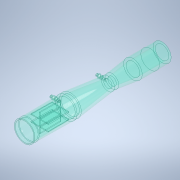
# Autodesk Inventor part: venturiwiwi
Saved by Autodesk Inventor 2020.2 (Build 242310000, 310)
## iProperties
Created: 2020-05-05
Part Number: venturiwiwi
Material: Generic
Document SubType Name: Modeling
Designer: JK
Density: 1 g/cm^3
Appearance: Indoor Pool
Author: JK
Autodesk Inventor part; units mm, degrees
sketch "Sketch1" plane through (0, 0, 0) normal (0, 1, 0) x (-1, 0, 0)
  line L0 (-5, 2.5) -> (5, 2.5)
  line L1 (5, 2.5) -> (5, -2.5)
  line L2 (5, -2.5) -> (-5, -2.5)
  line L3 (-5, -2.5) -> (-5, 2.5)
  line L4 (-5, 2.5) -> (5, -2.5) construction
  line L5 (5, 2.5) -> (-5, -2.5) construction
  line L6 (10.75, 52.5) -> (-10.75, 52.5)
  line L7 (-10.75, 52.5) -> (-10.75, 47.5)
  line L8 (-10.75, 47.5) -> (10.75, 47.5)
  line L9 (10.75, 47.5) -> (10.75, 52.5)
  line L10 (10.75, 52.5) -> (-10.75, 47.5) construction
  line L11 (-10.75, 52.5) -> (10.75, 47.5) construction
  line L12 (10.75, 47.5) -> (5, 2.5)
  line L13 (-10.75, 47.5) -> (-5, 2.5)
  line L14 (-13.75, 52.5) -> (13.75, 52.5)
  line L15 (13.75, 52.5) -> (13.75, 47.5)
  line L16 (13.75, 47.5) -> (-13.75, 47.5)
  line L17 (-13.75, 47.5) -> (-13.75, 52.5)
  line L18 (-13.75, 52.5) -> (13.75, 47.5) construction
  line L19 (13.75, 52.5) -> (-13.75, 47.5) construction
  line L20 (-8, 2.5) -> (8, 2.5)
  line L21 (8, 2.5) -> (8, -2.5)
  line L22 (8, -2.5) -> (-8, -2.5)
  line L23 (-8, -2.5) -> (-8, 2.5)
  line L24 (-8, 2.5) -> (8, -2.5) construction
  line L25 (8, 2.5) -> (-8, -2.5) construction
  line L26 (13.75, 47.5) -> (8, 2.5)
  line L27 (-13.75, 47.5) -> (-8, 2.5)
  line L28 (11.15, -27.5) -> (-11.15, -27.5)
  line L29 (-11.15, -27.5) -> (-11.15, -32.5)
  line L30 (-11.15, -32.5) -> (11.15, -32.5)
  line L31 (11.15, -32.5) -> (11.15, -27.5)
  line L32 (11.15, -27.5) -> (-11.15, -32.5) construction
  line L33 (-11.15, -27.5) -> (11.15, -32.5) construction
  line L34 (-8.15, -27.5) -> (8.15, -27.5)
  line L35 (8.15, -27.5) -> (8.15, -32.5)
  line L36 (8.15, -32.5) -> (-8.15, -32.5)
  line L37 (-8.15, -32.5) -> (-8.15, -27.5)
  line L38 (-8.15, -27.5) -> (8.15, -32.5) construction
  line L39 (8.15, -27.5) -> (-8.15, -32.5) construction
  line L40 (8, -2.5) -> (11.15, -27.5)
  line L41 (5, -2.5) -> (8.15, -27.5)
  line L42 (-5, -2.5) -> (-8.15, -27.5)
  line L43 (-8, -2.5) -> (-11.15, -27.5)
  line L44 (11.25, 102.5) -> (-11.25, 102.5)
  line L45 (-11.25, 102.5) -> (-11.25, 97.5)
  line L46 (-11.25, 97.5) -> (11.25, 97.5)
  line L47 (11.25, 97.5) -> (11.25, 102.5)
  line L48 (11.25, 102.5) -> (-11.25, 97.5) construction
  line L49 (-11.25, 102.5) -> (11.25, 97.5) construction
  line L50 (14.25, 102.5) -> (-14.25, 102.5)
  line L51 (-14.25, 102.5) -> (-14.25, 97.5)
  line L52 (-14.25, 97.5) -> (14.25, 97.5)
  line L53 (14.25, 97.5) -> (14.25, 102.5)
  line L54 (14.25, 102.5) -> (-14.25, 97.5) construction
  line L55 (-14.25, 102.5) -> (14.25, 97.5) construction
  line L56 (-11.25, 97.5) -> (-10.75, 52.5)
  line L57 (-14.25, 97.5) -> (-13.75, 52.5)
  line L58 (8.15, -57.5) -> (-8.15, -57.5)
  line L59 (-8.15, -57.5) -> (-8.15, -62.5)
  line L60 (-8.15, -62.5) -> (8.15, -62.5)
  line L61 (8.15, -62.5) -> (8.15, -57.5)
  line L62 (8.15, -57.5) -> (-8.15, -62.5) construction
  line L63 (-8.15, -57.5) -> (8.15, -62.5) construction
  line L64 (11.15, -57.5) -> (-11.15, -57.5)
  line L65 (-11.15, -57.5) -> (-11.15, -62.5)
  line L66 (-11.15, -62.5) -> (11.15, -62.5)
  line L67 (11.15, -62.5) -> (11.15, -57.5)
  line L68 (11.15, -57.5) -> (-11.15, -62.5) construction
  line L69 (-11.15, -57.5) -> (11.15, -62.5) construction
  line L70 (11.15, -32.5) -> (11.15, -57.5)
  line L71 (8.15, -32.5) -> (8.15, -57.5)
  line L72 (-8.15, -32.5) -> (-8.15, -57.5)
  line L73 (-11.15, -32.5) -> (-11.15, -57.5)
  line L74 (10.75, 52.5) -> (11.25, 97.5)
  line L75 (14.25, 97.5) -> (13.75, 52.5)
  line L76 (-12.5, 102.5) -> (12.5, 102.5)
  line L77 (12.5, 102.5) -> (12.5, 97.5)
  line L78 (12.5, 97.5) -> (-12.5, 97.5)
  line L79 (-12.5, 97.5) -> (-12.5, 102.5)
  line L80 (-12.5, 102.5) -> (12.5, 97.5) construction
  line L81 (12.5, 102.5) -> (-12.5, 97.5) construction
  line L82 (-13, 52.5) -> (13, 52.5)
  line L83 (13, 52.5) -> (13, 47.5)
  line L84 (13, 47.5) -> (-13, 47.5)
  line L85 (-13, 47.5) -> (-13, 52.5)
  line L86 (-13, 52.5) -> (13, 47.5) construction
  line L87 (13, 52.5) -> (-13, 47.5) construction
  line L88 (-12.5, 97.5) -> (-13, 52.5)
  line L89 (12.5, 97.5) -> (13, 52.5)
  line L90 (13, 47.5) -> (8, 2.5)
  line L91 (-13, 47.5) -> (-8, 2.5)
  line L92 (0, -95.5) -> (0, 135.5) projected
  point P0 (0, 0)
  point P1 (0, -30)
  point P2 (0, 100)
  point P3 (0, -60)
  point P4 (0, -60)
  point P5 (0, 0)
  point P6 (0, 100)
  point P7 (11.25, 97.5)
  point P8 (11.25, 97.5)
  point P9 (0, 50)
  point P10 (0, 100)
  point P11 (0, 100)
  point P12 (0, 50)
  point P13 (0, 50)
  point P14 (0, -60)
  point P15 (0, -30)
  dimension "d1" = 5
  dimension "d2" = 5
  dimension "d4" = 3
  dimension "d5" = 10
  dimension "d8" = 5
  dimension "d9" = 3
  dimension "d10" = 30
  dimension "d12" = 5
  dimension "d19" = 22.3
  dimension "d22" = 5
  dimension "d54" = 3
  dimension "d61" = 50
  dimension "d64" = 50
  dimension "d65" = 22.3
  dimension "d66" = 30
  dimension "d71" = 21.5
  dimension "d80" = 22.5
  dimension "d81" = 25
  dimension "d82" = 26
  constraints: 184 end point, 28 midpoint, 25 parallel, 12 horizontal, 12 perpendicular, 4 collinear, 4 point on line, 4 vertical alignment
  measures "d1" distance of L2.end L0.start
  measures "d2" distance of L8.end L6.start
  measures "d4" distance between parallel lines of L21 L1
  measures "d5" distance of L1.end L2.end
  measures "d8" distance of L34.end L35.end
  measures "d9" distance between parallel lines of L35 L31
  measures "d10" distance of point (0, -30) point (0, 0)
  measures "d12" distance of L46.end L44.start
  measures "d19" distance between parallel lines of L65 L67
  measures "d22" distance of L66.end L64.start
  measures "d54" distance between parallel lines of L7 L17
  measures "d61" distance of point (0, 50) point (0, 100)
  measures "d64" distance of point (0, 50) point (0, 0)
  measures "d65" distance between parallel lines of L29 L31
  measures "d66" distance of point (0, -60) point (0, -30)
  measures "d71" distance between parallel lines of L7 L9
  measures "d80" distance between parallel lines of L45 L47
  measures "d81" distance between parallel lines of L79 L77
  measures "d82" distance between parallel lines of L85 L83
revolve "Revolution1" add sketch "Sketch1" angle 360 about axis through (0, 0, -10) along (0, 0, 1) contours L20 L21 L22 L1 | L12 L16 L90 L20 | L22 L40 L28 L41 | L9 L14 L83 L16 | L28 L31 L30 L35 | L74 L52 L89 L14 | L30 L70 L64 L71 | L47 L50 L77 L52 | L64 L67 L66 L61
chamfer "Chamfer1" distance 0.25 angle 89 1 edges at (11.15, 0, -62.5) measured on face at (-9.9631, 1.5396, -62.5)
sketch "Sketch3" plane through (0, 0, 0) normal (1, 0, 0) x (0, 1, 0)
  circle A0 centre (0, 0) radius 0.75
  circle A1 centre (0, 50) radius 0.75
  line L0 (12.5, 102.5) -> (-12.5, 102.5) projected
  dimension "d30" = 1.5
  dimension "d31" = 1.5
  dimension "d83" = 52.5
  constraints: 2 centre point, 1 coincident, 1 vertical alignment
  measures "d30" diameter of A0
  measures "d31" diameter of A1
  measures "d83" distance from line of L0 A1.centre
extrude "Extrusion1" cut sketch "Sketch3" against normal blind 56.5
ref_plane "Work Plane2" through (-13, 0, 50) normal (1, 0, 0) x (0, 1, 0)
sketch "Sketch6" plane through (-13, 0, 50) normal (1, 0, 0) x (0, 1, 0)
  circle A0 centre (0, 0) radius 0.75
  circle A1 centre (0, 0) radius 1.5
  line L0 (12.5, 52.5) -> (-12.5, 52.5) projected
  point P0 (-0.75, -50)
  dimension "d35" = 1.5
  dimension "d36" = 3
  dimension "d84" = 52.5
  constraints: 2 centre point, 1 concentric
  measures "d35" diameter of A0
  measures "d36" diameter of A1
  measures "d84" distance from line of L0 A0.centre
extrude "Extrusion2" add sketch "Sketch6" along normal blind 1.5 and the other way blind 8
ref_plane "Work Plane3" through (-8, 0, 0) normal (1, 0, 0) x (0, 1, 0)
sketch "Sketch7" plane through (-8, 0, 0) normal (1, 0, 0) x (0, 1, 0)
  circle A0 centre (0, 0) radius 0.75
  circle A1 centre (0, 0) radius 1.5
  point P0 (0, 0)
  dimension "d43" = 1.5
  dimension "d44" = 3
  constraints: 2 centre point, 2 coincident
  measures "d43" diameter of A0
  measures "d44" diameter of A1
extrude "Extrusion3" add sketch "Sketch7" along normal blind 2 and the other way blind 8
fillet "Fillet1" radius 1 6 edges at (-10.7238, -0.75, 50) (-10.736, 0.5491, 49.4892) (-10.7359, 0.5509, 50.5089) (-4.9434, -0.75, 0) (-4.9698, 0.5484, -0.5116) (-4.9696, 0.5501, 0.5098)
sketch "Sketch8" plane through (0, 0, 0) normal (0, 1, 0) x (-1, 0, 0)
  line L0 (21, 48.5) -> (21, 51.5) projected
  line L1 (21, 51.5) -> (18, 52.25)
  line L2 (18, 52.25) -> (18, 51.5)
  line L3 (18, 51.5) -> (15, 52.25)
  line L4 (15, 52.25) -> (15, 51.5)
  line L5 (15, 51.5) -> (21, 51.5)
  line L6 (15.3366, 50) -> (24.3627, 50)
  line L7 (21, 48.5) -> (13, 48.5) projected
  point P0 (0, 0)
  dimension "d50" = 0.75
  dimension "d51" = 3
  dimension "d52" = 3
  dimension "d55" = 1.5
  constraints: 12 end point, 2 parallel, 1 horizontal, 1 horizontal alignment, 1 midpoint, 1 perpendicular
  measures "d50" distance of L1.end L2.end
  measures "d51" distance from line of L0 L2.end
  measures "d52" distance from line of L2.end L4
  measures "d55" distance between parallel lines of L7 L6
revolve "Revolution2" add sketch "Sketch8" angle 360 about axis through (-15.3366, 0, 50) along (-1, 0, 0)
sketch "Sketch9" plane through (0, 0, 0) normal (0, 1, 0) x (-1, 0, 0)
  line L0 (16, -1.5) -> (16, 1.5) projected
  line L1 (16, 1.5) -> (13, 2.25)
  line L2 (13, 2.25) -> (13, 1.5)
  line L3 (16, 1.5) -> (8, 1.5) projected
  line L4 (13, 1.5) -> (10, 2.25)
  line L5 (10, 2.25) -> (10, 1.5)
  line L6 (10, 1.5) -> (16, 1.5)
  line L7 (16, 0) -> (10.3652, 0)
  line L8 (10.3652, 0) -> (16.7682, 0)
  point P0 (0, 0)
  point P1 (10, 1.5)
  dimension "d56" = 0.75
  dimension "d57" = 3
  dimension "d58" = 3
  constraints: 14 end point, 2 point on line, 1 horizontal, 1 horizontal alignment, 1 parallel, 1 perpendicular, 1 vertical
  measures "d56" distance of L2.end L1.end
  measures "d57" distance of L2.end L5.end
  measures "d58" distance of L3.start L2.end
revolve "Revolution3" add sketch "Sketch9" angle 360 about axis through (-10.3652, 0, 0) along (-1, 0, 0)
fillet "Fillet2" radius 0.5 2 edges at (-16, 0, -1.5) (-21, 0, 48.5)
ref_plane "Work Plane4" through (0, 0, 84.5) normal (0, 0, 1) x (1, 0, 0)
sketch "Sketch14" plane through (0, 0, 84.5) normal (0, 0, 1) x (1, 0, 0)
  line L0 (11.25, -0.5) -> (-11.25, 0.5) construction
  line L1 (-11.25, -0.5) -> (11.25, 0.5) construction
  line L2 (-0.5, -11.25) -> (0.5, -11.25)
  line L3 (0.5, -11.25) -> (0.5, 11.25)
  line L4 (0.5, 11.25) -> (-0.5, 11.25)
  line L5 (-0.5, 11.25) -> (-0.5, -11.25)
  line L6 (-0.5, -11.25) -> (0.5, 11.25) construction
  line L7 (0.5, -11.25) -> (-0.5, 11.25) construction
  circle A0 centre (0, 0) radius 11.25 projected
  circle A1 centre (0, 0) radius 11.25 projected
  line L8 (10.5915, -4.4997) -> (-10.6918, -4.4997)
  line L9 (-10.6918, -4.4997) -> (-10.6918, -3.4997)
  line L10 (-10.6918, -3.4997) -> (10.5915, -3.4997)
  line L11 (10.5915, -3.4997) -> (10.5915, -4.4997)
  line L12 (10.5915, -4.4997) -> (-10.6918, -3.4997) construction
  line L13 (-10.6918, -4.4997) -> (10.5915, -3.4997) construction
  line L14 (10.5915, 4.4997) -> (-10.6918, 4.4997)
  line L15 (-10.6918, 4.4997) -> (-10.6918, 3.4997)
  line L16 (-10.6918, 3.4997) -> (10.5915, 3.4997)
  line L17 (10.5915, 3.4997) -> (10.5915, 4.4997)
  line L18 (10.5915, 4.4997) -> (-10.6918, 3.4997) construction
  line L19 (-10.6918, 4.4997) -> (10.5915, 3.4997) construction
  point P0 (0.5, 11.2389)
  point P1 (-0.5, 11.2389)
  point P2 (-0.5, -11.2389)
  point P3 (0.5, -11.2389)
  point P4 (-0.0502, -3.9997)
  point P5 (-0.0502, 3.9997)
  point P6 (-0.0502, 3.9997)
  point P7 (-0.0502, -3.9997)
  point P8 (0, -11.25)
  point P9 (0, 11.25)
  point P10 (-0.5, -3.4997)
  point P11 (-0.5, -4.4997)
  point P12 (0.5, -3.4997)
  point P13 (0.5, -4.4997)
  point P14 (10.5915, 3.7925)
  point P15 (10.3109, 4.4997)
  point P16 (0.5, 4.4997)
  point P17 (0.5, 3.4997)
  point P18 (-0.5, 3.4997)
  point P19 (-0.5, 4.4997)
  point P20 (-10.3109, 4.4997)
  dimension "d92" = 1
  dimension "d100" = 1
  dimension "d101" = 1
  dimension "d102" = 4
  dimension "d103" = 4
  constraints: 40 end point, 10 midpoint, 6 parallel, 3 horizontal, 3 perpendicular, 2 point on circle, 1 tangent, 1 vertical alignment
  measures "d92" distance between parallel lines of L5 L3
  measures "d100" distance between parallel lines of L10 L8
  measures "d101" distance between parallel lines of L14 L16
  measures "d102" distance of point (-0.05, -4) point (0, 0)
  measures "d103" distance of A0.centre point (-0.05, 4)
extrude "Extrusion6" add sketch "Sketch14" against normal blind 25 contours A0 L5 L8 L3 | L8 A0 L10 L5 | L5 L10 L3 L8 | L8 L9 A0 | L3 L10 L11 A0 L8 | A0 L11 L8 | L5 L16 L3 L10 | L16 A0 L14 L5 | L5 L14 L3 L16 | L3 L14 A0 L17 L16 | L5 A0 L3 L14 | L5 L4 A0 | A0 L4 L3
sketch "Sketch11" plane through (0, 0, 0) normal (0, 1, 0) x (-1, 0, 0)
  line L0 (10.75, 52.5) -> (10.75, 47.5) projected
  line L1 (10.75, 201.4514) -> (11.25, 82.5)
  line L2 (-11.25, 82.5) -> (-12.405, 201.4514)
  line L3 (-11.25, 97.5) -> (-10.75, 52.5) projected
  line L4 (11.25, 82.5) -> (10.75, 201.4514)
  line L5 (-12.405, 201.4514) -> (10.75, 201.4514)
  line L6 (12.75, 52.5) -> (-12.75, 52.5) projected
  line L7 (11.25, 102.5) -> (-11.25, 102.5) projected
  line L8 (0, 82.5) -> (0, 52.5)
  line L9 (-11.25, 82.5) -> (11.25, 82.5) projected
  line L10 (0, 82.5) -> (11.25, 82.5)
  point P0 (0, 0)
  point P1 (-11.25, 102.5)
  constraints: 12 end point, 2 horizontal, 2 point on line, 1 collinear, 5 other
body "Solid1"
